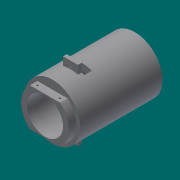
# Autodesk Inventor part: 知能ロボコン吸引部２.1
Saved by Autodesk Inventor 2013 (Build 170138000, 138)
## iProperties
Created: 2014-11-21
Part Number: 知能ロボコン吸引部２.1
Material: 一般
Document SubType Name: Modeling
Designer: horumo136
Density: 1 g/cm^3
Author: horumo136
Autodesk Inventor part; units mm, degrees
ref_plane "YZ Plane" through (0, 0, 0) normal (1, 0, 0) x (0, 1, 0)
sketch "スケッチ1" plane through (0, 0, 0) normal (0, 0, 1) x (1, 0, 0)
  line L0 (0, 0) -> (32, 0)
  line L1 (0, 0) -> (0, 30)
  line L2 (0, 30) -> (35, 30)
  line L3 (35, 30) -> (32, 0)
  line L4 (32, 0) -> (33.990074, -0.199007)
  line L5 (33.990074, -0.199007) -> (36.990074, 29.800993)
  line L6 (36.990074, 29.800993) -> (35, 30)
  line L7 (0, 0) -> (0, -80)
  line L8 (0, -80) -> (26.009975, -80)
  line L9 (32, 0) -> (24.019901, -79.800993)
  line L10 (33.990074, -0.199007) -> (26.009975, -80)
  line L11 (26.009975, -80) -> (24.019901, -79.800993)
  line L12 (26.009975, -80) -> (36.990074, -80)
  line L13 (36.990074, -80) -> (36.990074, 29.800993)
  line L14 (24.019901, -79.800993) -> (24, -80)
  dimension "d0" = 32
  dimension "d1" = 30
  dimension "d2" = 35
  dimension "d3" = 2
  dimension "d4" = 80
  constraints: 30 end point, 10 perpendicular, 2 parallel, 1 collinear, 1 horizontal, 1 point on line
  measures "d0" distance of L0.start L0.end
  measures "d1" distance of L0.start L1.end
  measures "d2" distance of L1.end L2.end
  measures "d3" distance of L0.end L4.end
  measures "d4" distance of L0.start L7.end
revolve "回転1" add sketch "スケッチ1" angle 360 about axis through (0, 0, 0) along (0, 1, 0) contours L3 L6 L5 L4 | L4 L10 L11 L9 | L5 L13 L12 L10 | L11 L8 L14
ref_plane "作業平面4" through (0, 0, 37) normal (0, 0, 1) x (1, 0, 0)
sketch "スケッチ2" plane through (0, 0, 37) normal (0, 0, 1) x (1, 0, 0)
  circle A0 centre (0, 0) radius 33
  line L0 (0, 0) -> (0, -46)
  line L1 (-13.5, -41) -> (13.5, -41)
  line L2 (13.5, -41) -> (13.5, -51)
  line L3 (13.5, -51) -> (-13.5, -51)
  line L4 (-13.5, -51) -> (-13.5, -41)
  line L5 (-13.5, -41) -> (13.5, -51) construction
  line L6 (13.5, -41) -> (-13.5, -51) construction
  dimension "d10" = 66
  dimension "d11" = 46
  dimension "d12" = 27
  dimension "d13" = 10
  constraints: 14 end point, 2 midpoint, 2 parallel, 1 centre point, 1 coincident, 1 horizontal, 1 perpendicular, 1 vertical
  measures "d10" diameter of A0
  measures "d11" distance of L0.start L0.end
  measures "d12" distance of L2.end L3.end
  measures "d13" distance of L1.end L2.end
sketch "スケッチ4" plane through (0, -80, 0) normal (0, -1, 0) x (1, 0, 0)
  circle A0 centre (0, 0) radius 36.990074
  line L0 (-20, 25.4) -> (20, 25.4)
  line L1 (20, 25.4) -> (20, -25.4)
  line L2 (20, -25.4) -> (-20, -25.4)
  line L3 (-20, -25.4) -> (-20, 25.4)
  line L4 (-20, 25.4) -> (20, -25.4) construction
  line L5 (20, 25.4) -> (-20, -25.4) construction
  arc A1 (20, 13.280835) -> (-20, 13.280835) centre (0, 0) ccw
  arc A2 (-20, -13.280835) -> (20, -13.082614) centre (-0.064724, -0.120675) ccw
  dimension "d14" = 40
  dimension "d15" = 50.8
  constraints: 12 end point, 4 point on circle, 4 point on line, 2 centre point, 2 midpoint, 2 parallel, 1 concentric, 1 horizontal, 1 perpendicular
  measures "d14" distance of L1.end L2.end
  measures "d15" distance of L0.end L1.end
extrude "押し出し1" add sketch "スケッチ4" along normal blind 10 contours L0 L1 A1 L3 | A2 L1 L2 L3
sketch "スケッチ5" plane through (-20, -80, 25.4) normal (0, 0, 1) x (1, 0, 0)
  line L0 (0, 0) -> (40, 0) projected
  line L1 (40, 0) -> (40, -10) projected
  line L2 (20, 0) -> (20, -5)
  line L3 (20, -5) -> (35, -5)
  line L4 (20, -5) -> (5, -5)
  circle A0 centre (5, -5) radius 1.25
  circle A1 centre (35, -5) radius 1.25
  point P0 (20, 80)
  dimension "d18" = 5
  dimension "d19" = 15
  dimension "d20" = 15
  dimension "d21" = 2.5
  dimension "d22" = 2.5
  constraints: 6 end point, 2 centre point, 2 coincident, 1 collinear, 1 midpoint, 1 parallel, 1 perpendicular
  measures "d18" distance of L2.start L2.end
  measures "d19" distance of L2.end L3.end
  measures "d20" distance of L2.end L4.end
  measures "d21" diameter of A0
  measures "d22" diameter of A1
extrude "押し出し2" cut sketch "スケッチ5" against normal blind 51
extrude "押し出し3" cut sketch "スケッチ2" against normal blind 80 contours L1 L2 L3 L4
sketch "スケッチ6" plane through (0, -80, 0) normal (0, -1, 0) x (1, 0, 0)
  arc A0 (-20, -13.280835) -> (2.651317, -23.853103) centre (-0.064724, -0.120675) ccw
  arc A1 (20, -13.266499) -> (2.651317, -23.853103) centre (0, 0) ccw
  line L0 (20, -13.266499) -> (20, -25.4)
  line L1 (-20, -25.4) -> (-20, -13.280835)
  line L2 (20, 25.4) -> (20, 13.280835)
  arc A2 (20, 13.280835) -> (-20, 13.280835) centre (0, 0) ccw
  line L3 (-20, 13.280835) -> (-20, 25.4)
  arc A3 (-20, 13.280835) -> (-20, -13.280835) centre (0.118076, 0) ccw
  arc A4 (-20, 25.4) -> (-20, -25.4) centre (1.067511, 0) ccw
  arc A5 (20, -13.266499) -> (20, 13.280835) centre (0.010794, 0.007168) ccw
  arc A6 (20, -25.4) -> (20, 25.4) centre (-1.067511, 0) ccw
  dimension "d27" = 33
  dimension "d28" = 33
  constraints: 8 point on circle, 4 centre point, 2 tangent
  measures "d27" radius of A4
  measures "d28" radius of A6
sketch "スケッチ6 outline for 押し出し4" plane through (0, -80, 0) normal (0, -1, 0) x (1, 0, 0)
  line L0 (20, 25.4) -> (20, 13.280835)
  arc A0 (20, 13.280835) -> (-20, 13.280835) centre (0, 0) ccw
  line L1 (-20, 13.280835) -> (-20, 25.4)
  arc A1 (-20, 25.4) -> (-20, -25.4) centre (1.067511, 0) ccw
  line L2 (-20, -25.4) -> (-20, -13.280835)
  arc A2 (-20, -13.280835) -> (2.651317, -23.853103) centre (-0.064724, -0.120675) ccw
  arc A3 (2.651317, -23.853103) -> (20, -13.266499) centre (0, 0) cw
  line L3 (20, -13.266499) -> (20, -25.4)
  arc A4 (20, -25.4) -> (20, 25.4) centre (-1.067511, 0) ccw
extrude "押し出し4" add sketch "スケッチ6 outline for 押し出し4" along normal blind 10
sketch "スケッチ7" plane through (0, -51, 0) normal (0, 1, 0) x (1, 0, 0)
  arc A0 (13.5, 34.438577) -> (-13.5, 34.438577) centre (0, 0) ccw
  line L0 (-10, 26.990074) -> (10, 26.990074)
  line L1 (10, 26.990074) -> (10, 46.990074)
  line L2 (10, 46.990074) -> (-10, 46.990074)
  line L3 (-10, 46.990074) -> (-10, 26.990074)
  line L4 (-10, 26.990074) -> (10, 46.990074) construction
  line L5 (10, 26.990074) -> (-10, 46.990074) construction
  point P0 (0, 36.990074)
  dimension "d31" = 20
  constraints: 12 end point, 2 midpoint, 2 parallel, 1 horizontal, 1 perpendicular, 1 point on circle
  measures "d31" distance of L1.end L0.end
extrude "押し出し5" add sketch "スケッチ7" against normal blind 5
mirror "ミラー1" about plane through (0, 0, 0) normal (0, 0, 1) of "押し出し5"
ref_plane "作業平面5" through (10, -51, 41.301396) normal (0, 1, 0) x (1, 0, 0)
sketch "スケッチ8" plane through (10, -51, 41.301396) normal (0, 1, 0) x (1, 0, 0)
  line L0 (-14.976748, 1.255042) -> (-4.976748, 1.255042)
  line L1 (-4.976748, 1.255042) -> (-4.976748, 81.255042)
  line L2 (-4.976748, 81.255042) -> (-14.976748, 81.255042)
  line L3 (-14.976748, 81.255042) -> (-14.976748, 1.255042)
  line L4 (-14.976748, 1.255042) -> (-4.976748, 81.255042) construction
  line L5 (-4.976748, 1.255042) -> (-14.976748, 81.255042) construction
  line L6 (-9.976748, 81.255042) -> (-9.976748, 1.255042)
  circle A0 centre (-9.976748, 81.255042) radius 1
  circle A1 centre (-9.976748, 1.255042) radius 1
  point P0 (-9.976748, 41.255042)
  dimension "d42" = 10
  dimension "d43" = 80
  dimension "d44" = 2
  dimension "d45" = 2
  constraints: 14 end point, 4 midpoint, 2 centre point, 2 coincident, 2 parallel, 1 horizontal, 1 perpendicular
  measures "d42" distance of L2.end L1.end
  measures "d43" distance of L1.end L0.end
  measures "d44" diameter of A0
  measures "d45" diameter of A1
extrude "押し出し7" cut sketch "スケッチ8" against normal blind 5 contours L6 A1 L0 | L0 A1 | L0 A1 L6 | A0 L2 L6 | L6 L2 A0 | L2 A0
